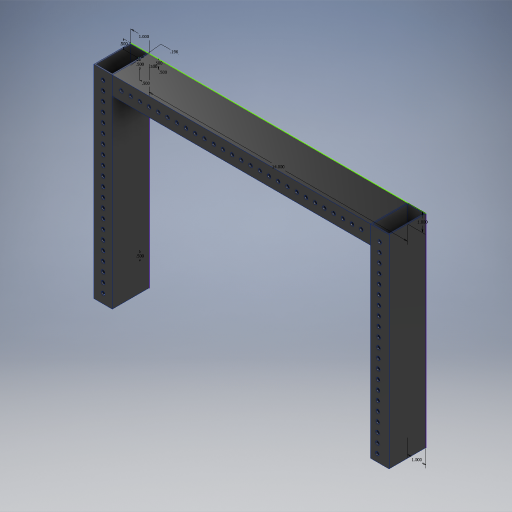
# Autodesk Inventor part: 2024-220-000-Hard-Stop
Saved by Autodesk Inventor 2024.2 (Build 282272000, 272)
## iProperties
Created: 2024-01-23
Part Number: 2024-220-000-Hard-Stop
Material: Aluminum 6061
Document SubType Name: Modeling
Designer: rohan
Density: 2.7 g/cm^3
Appearance: Aluminum - Flat
Author: rohan
Autodesk Inventor part; units mm, degrees
ref_plane "YZ Plane" through (0, 0, 0) normal (1, 0, 0) x (0, 1, 0)
ref_plane "XZ Plane" through (0, 0, 0) normal (0, 1, 0) x (-1, 0, 0)
ref_plane "XY Plane" through (0, 0, 0) normal (0, 0, 1) x (1, 0, 0)
sketch "Sketch1" plane through (0, 0, 0) normal (0, 0, 1) x (1, 0, 0)
  line L0 (0, 0) -> (25.4, 0)
  line L1 (25.4, 0) -> (25.4, 279.4)
  line L2 (25.4, 279.4) -> (0, 279.4)
  line L3 (0, 279.4) -> (0, 0)
  line L4 (25.4, 279.4) -> (381, 279.4)
  line L5 (381, 279.4) -> (381, 254)
  line L6 (381, 254) -> (25.4, 254)
  line L7 (25.4, 254) -> (25.4, 279.4)
  line L8 (381, 279.4) -> (406.4, 279.4)
  line L9 (406.4, 279.4) -> (406.4, 0)
  line L10 (406.4, 0) -> (381, 0)
  line L11 (381, 0) -> (381, 279.4)
  circle A0 centre (12.7, 266.7) radius 2.4892
  circle A1 centre (38.1, 266.7) radius 2.4892
  circle A2 centre (12.7, 254) radius 2.4892
  circle A3 centre (12.7, 241.3) radius 2.4892
  circle A4 centre (12.7, 228.6) radius 2.4892
  circle A5 centre (12.7, 215.9) radius 2.4892
  circle A6 centre (12.7, 203.2) radius 2.4892
  circle A7 centre (12.7, 190.5) radius 2.4892
  circle A8 centre (12.7, 177.8) radius 2.4892
  circle A9 centre (12.7, 165.1) radius 2.4892
  circle A10 centre (12.7, 152.4) radius 2.4892
  circle A11 centre (12.7, 139.7) radius 2.4892
  circle A12 centre (12.7, 127) radius 2.4892
  circle A13 centre (12.7, 114.3) radius 2.4892
  circle A14 centre (12.7, 101.6) radius 2.4892
  circle A15 centre (12.7, 88.9) radius 2.4892
  circle A16 centre (12.7, 76.2) radius 2.4892
  circle A17 centre (12.7, 63.5) radius 2.4892
  circle A18 centre (12.7, 50.8) radius 2.4892
  circle A19 centre (12.7, 38.1) radius 2.4892
  circle A20 centre (12.7, 25.4) radius 2.4892
  circle A21 centre (12.7, 12.7) radius 2.4892
  circle A22 centre (393.5275, 264.3341) radius 2.4892
  circle A23 centre (393.3697, 251.6351) radius 2.4892
  circle A24 centre (393.2119, 238.936) radius 2.4892
  circle A25 centre (393.0541, 226.237) radius 2.4892
  circle A26 centre (392.8963, 213.538) radius 2.4892
  circle A27 centre (392.7385, 200.839) radius 2.4892
  circle A28 centre (392.5807, 188.14) radius 2.4892
  circle A29 centre (392.4229, 175.4409) radius 2.4892
  circle A30 centre (392.2652, 162.7419) radius 2.4892
  circle A31 centre (392.1074, 150.0429) radius 2.4892
  circle A32 centre (391.9496, 137.3439) radius 2.4892
  circle A33 centre (391.7918, 124.6449) radius 2.4892
  circle A34 centre (391.634, 111.9458) radius 2.4892
  circle A35 centre (391.4762, 99.2468) radius 2.4892
  circle A36 centre (391.3184, 86.5478) radius 2.4892
  circle A37 centre (391.1606, 73.8488) radius 2.4892
  circle A38 centre (391.0028, 61.1498) radius 2.4892
  circle A39 centre (390.845, 48.4507) radius 2.4892
  circle A40 centre (390.6872, 35.7517) radius 2.4892
  circle A41 centre (390.5294, 23.0527) radius 2.4892
  circle A42 centre (390.3716, 10.3537) radius 2.4892
  circle A43 centre (50.8, 266.7) radius 2.4892
  circle A44 centre (63.5, 266.7) radius 2.4892
  circle A45 centre (76.2, 266.7) radius 2.4892
  circle A46 centre (88.9, 266.7) radius 2.4892
  circle A47 centre (101.6, 266.7) radius 2.4892
  circle A48 centre (114.3, 266.7) radius 2.4892
  circle A49 centre (127, 266.7) radius 2.4892
  circle A50 centre (139.7, 266.7) radius 2.4892
  circle A51 centre (152.4, 266.7) radius 2.4892
  circle A52 centre (165.1, 266.7) radius 2.4892
  circle A53 centre (177.8, 266.7) radius 2.4892
  circle A54 centre (190.5, 266.7) radius 2.4892
  circle A55 centre (203.2, 266.7) radius 2.4892
  circle A56 centre (215.9, 266.7) radius 2.4892
  circle A57 centre (228.6, 266.7) radius 2.4892
  circle A58 centre (241.3, 266.7) radius 2.4892
  circle A59 centre (254, 266.7) radius 2.4892
  circle A60 centre (266.7, 266.7) radius 2.4892
  circle A61 centre (279.4, 266.7) radius 2.4892
  circle A62 centre (292.1, 266.7) radius 2.4892
  circle A63 centre (304.8, 266.7) radius 2.4892
  circle A64 centre (317.5, 266.7) radius 2.4892
  circle A65 centre (330.2, 266.7) radius 2.4892
  circle A66 centre (342.9, 266.7) radius 2.4892
  circle A67 centre (355.6, 266.7) radius 2.4892
  circle A68 centre (368.3, 266.7) radius 2.4892
  point P0 (25.4, 266.7)
  point P1 (25.4, 254)
  dimension "d0" = 25.4
  dimension "d2" = 355.6
  dimension "d3" = 25.4
  dimension "d4" = 25.4
  dimension "d5" = 4.9784
  dimension "d8" = 12.7
  dimension "d9" = 12.7
  dimension "d12" = 12.7
  dimension "d26" = 12.7
  dimension "d64" = 12.7
  dimension "d65" = 12.7
  dimension "d68" = 12.7
  constraints: 69 centre point, 24 end point, 6 parallel, 4 horizontal, 3 perpendicular, 2 vertical, 1 midpoint, 1 point on line, 92 other
  measures "d0" distance of L2.end L1.end
  measures "d2" distance of L5.end L6.end
  measures "d3" distance of L4.end L5.end
  measures "d4" distance of L9.end L10.end
  measures "d5" diameter of A0
  measures "d8" distance from line of L2 A0.centre
  measures "d9" distance of point (25.4, 266.7) A0.centre
  measures "d12" distance of A0.centre A2.centre
  measures "d26" distance of A19.centre A20.centre
  measures "d64" distance from line of L7 A1.centre
  measures "d65" distance from line of L4 A1.centre
  measures "d68" distance of A1.centre A43.centre
extrude "Extrusion1" add sketch "Sketch1" along normal blind 50.8 contours L3 L2 L1 L0
extrude "Extrusion2" add sketch "Sketch1" along normal blind 50.8 separate body contours L1 L4 L5 L6
extrude "Extrusion3" add sketch "Sketch1" along normal blind 50.8 separate body contours L5 L8 L9 L10 L11
sketch "Sketch2" plane through (0, 279.4, 0) normal (0, 1, 0) x (1, 0, 0)
  line L0 (25.4, 0) -> (0, 0) projected
  line L1 (0, 0) -> (0, -50.8) projected
  line L2 (25.4, -50.8) -> (0, -50.8) projected
  line L3 (25.4, 0) -> (25.4, -50.8) projected
  line L4 (23.8125, -49.2125) -> (1.5875, -49.2125)
  line L5 (1.5875, -49.2125) -> (1.5875, -1.5875)
  line L6 (1.5875, -1.5875) -> (23.8125, -1.5875)
  line L7 (23.8125, -1.5875) -> (23.8125, -49.2125)
  point P0 (0, 0)
  dimension "d38" = 1.5875
  constraints: 8 end point, 3 other
  measures "d38" distance between parallel lines of L3 L7
extrude "Extrusion4" cut sketch "Sketch2" against normal blind 322.2625 contours L4 L5 L6 L7 bodies 1
sketch "Sketch3" plane through (381, 279.4, 0) normal (0, 1, 0) x (1, 0, 0)
  line L0 (25.4, 0) -> (0, 0) projected
  line L1 (0, 0) -> (0, -50.8) projected
  line L2 (25.4, -50.8) -> (0, -50.8) projected
  line L3 (25.4, 0) -> (25.4, -50.8) projected
  line L4 (23.8125, -49.2125) -> (1.5875, -49.2125)
  line L5 (1.5875, -49.2125) -> (1.5875, -1.5875)
  line L6 (1.5875, -1.5875) -> (23.8125, -1.5875)
  line L7 (23.8125, -1.5875) -> (23.8125, -49.2125)
  point P0 (-381, 0)
  dimension "d41" = 1.5875
  constraints: 8 end point, 3 other
  measures "d41" distance between parallel lines of L3 L7
extrude "Extrusion5" cut sketch "Sketch3" against normal blind 322.2625 contours L4 L5 L6 L7 bodies 3
sketch "Sketch4" plane through (381, 254, 0) normal (1, 0, 0) x (0, 0, -1)
  line L0 (0, 0) -> (0, 25.4) projected
  line L1 (0, 25.4) -> (-50.8, 25.4) projected
  line L2 (-50.8, 0) -> (-50.8, 25.4) projected
  line L3 (0, 0) -> (-50.8, 0) projected
  line L4 (-49.2125, 23.8125) -> (-1.5875, 23.8125)
  line L5 (-1.5875, 23.8125) -> (-1.5875, 1.5875)
  line L6 (-1.5875, 1.5875) -> (-49.2125, 1.5875)
  line L7 (-49.2125, 1.5875) -> (-49.2125, 23.8125)
  point P0 (0, -254)
  dimension "d44" = 1.5875
  constraints: 8 end point, 3 other
  measures "d44" distance between parallel lines of L2 L7
extrude "Extrusion6" cut sketch "Sketch4" against normal blind 279.4 contours L4 L5 L6 L7 bodies 2
sketch "Sketch5" plane through (25.4, 254, 0) normal (-1, 0, 0) x (0, 0, 1)
  line L0 (0, 25.4) -> (0, 0) projected
  line L1 (0, 0) -> (50.8, 0) projected
  line L2 (50.8, 25.4) -> (50.8, 0) projected
  line L3 (0, 25.4) -> (50.8, 25.4) projected
  line L4 (49.2125, 23.8125) -> (49.2125, 1.5875)
  line L5 (49.2125, 1.5875) -> (1.5875, 1.5875)
  line L6 (1.5875, 1.5875) -> (1.5875, 23.8125)
  line L7 (1.5875, 23.8125) -> (49.2125, 23.8125)
  point P0 (0, -254)
  dimension "d54" = 1.5875
  constraints: 8 end point, 3 other
  measures "d54" distance between parallel lines of L3 L7
extrude "Extrusion7" cut sketch "Sketch5" against normal blind 119.0625 contours L4 L5 L6 L7 bodies 2
